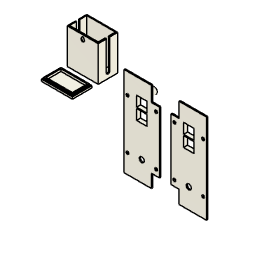
AP Panels (Autodesk Fusion 360 design; units mm, degrees)
Autodesk Fusion 360 part; units mm, degrees
sketch "Main" plane through (0, 0, 0) normal (0, 1, 0) x (1, 0, 0) in component "Front Left Plate"
  line L0 (-12, -11) -> (-12, 145)
  line L1 (-12, 145) -> (36, 145)
  line L2 (36, 145) -> (36, 122)
  line L3 (36, 122) -> (50, 122)
  line L4 (50, 122) -> (50, 15)
  line L5 (50, 15) -> (36, 15)
  line L6 (36, 15) -> (36, -11)
  line L7 (36, -11) -> (-12, -11)
  line L8 (-12, 0) -> (0, 0) construction
  line L9 (0, 0) -> (38, 0) construction
  line L10 (19, 145) -> (19, 139) construction
  line L11 (0, 139) -> (38, 139) construction
  line L12 (0, 139) -> (0, 0) construction
  line L13 (38, 139) -> (38, 0) construction
  line L14 (19, 139) -> (19, 0) construction
  circle A0 centre (-6, 25) radius 2.5
  line L15 (-6, 0) -> (-6, 139) construction
  line L16 (0, 139) -> (-12, 139) construction
  line L17 (36, 15) -> (-12, 15) construction
  line L18 (36, 122) -> (-12, 122) construction
  circle A1 centre (-6, 112) radius 2.5
  circle A2 centre (44, 25) radius 2.5
  circle A3 centre (44, 112) radius 2.5
  circle A4 centre (19, 110) radius 4.5
  line L19 (28, 55) -> (10, 55)
  line L20 (10, 55) -> (10, 37)
  line L21 (10, 37) -> (28, 37)
  line L22 (28, 37) -> (28, 55)
  line L23 (28, 55) -> (10, 37) construction
  line L24 (10, 55) -> (28, 37) construction
  line L25 (28, 35) -> (10, 35)
  line L26 (10, 35) -> (10, 17)
  line L27 (10, 17) -> (28, 17)
  line L28 (28, 17) -> (28, 35)
  line L29 (28, 35) -> (10, 17) construction
  line L30 (10, 35) -> (28, 17) construction
  point P0 (19, 46)
  point P1 (19, 26)
  dimension "d3" = 156
  dimension "d7" = 48
  dimension "d8" = 62
  dimension "d9" = 23
  dimension "d12" = 12
  dimension "d13" = 11
  dimension "d15" = 6
  dimension "d16" = 38
  dimension "d17" = 107
  dimension "d18" = 5
  dimension "d19" = 10
  dimension "d20" = 5
  dimension "d21" = 5
  dimension "d22" = 10
  dimension "d23" = 6
  dimension "d25" = 10
  dimension "d27" = 5
  dimension "d28" = 6
  dimension "d29" = 10
  dimension "d32" = 9
  dimension "d33" = 35
  dimension "d35" = 18
  dimension "d36" = 55
  dimension "d37" = 2
  constraint vertical L0
  constraint perpendicular L0 L1
  constraint perpendicular L2 L3
  constraint perpendicular L3 L4
  constraint perpendicular L4 L5
  constraint perpendicular L5 L6
  constraint horizontal L7
  constraint equal L1 L7
  constraint coincident L0 L8.start
  constraint perpendicular L0 L8
  constraint coincident L8.end L9.start
  constraint coincident L1 L10.start
  constraint perpendicular L1 L10
  constraint perpendicular L2 L11
  constraint midpoint L10.end L11
  constraint vertical L12
  constraint horizontal L9
  constraint equal L9 L11
  constraint midpoint L9 L14.end
  constraint midpoint L8 L15.start
  constraint perpendicular L8 L15
  constraint coincident L0 L16.end
  constraint perpendicular L0 L16
  constraint coincident L15.end L16
  constraint coincident A0.centre L15
  constraint coincident L0 L17.end
  constraint perpendicular L0 L17
  constraint coincident L0 L18.end
  constraint perpendicular L0 L18
  constraint coincident L15 A1.centre
  constraint coincident L14 A4.centre
  constraint horizontal L19
  constraint perpendicular L19 L20
  constraint parallel L19 L21
  constraint parallel L20 L22
  constraint coincident L23 P0
  constraint coincident L24 P0
  constraint coincident L14 P0
  constraint equal L19 L22
  constraint horizontal L25
  constraint perpendicular L25 L26
  constraint parallel L25 L27
  constraint parallel L26 L28
  constraint coincident L29 P1
  constraint coincident L30 P1
  constraint equal L22 L28
  constraint equal L22 L25
  constraint coincident L14 P1
  measures "d3" distance of L0.start L0.end
  measures "d7" distance of L0.end L1.end
  measures "d8" distance of L0 L4
  measures "d9" distance of L1.end L2.end
  measures "d12" distance of L8.start L8.end
  measures "d13" distance of L7 L8.end
  measures "d16" distance of L8.end L9.end
  measures "d17" distance of L3.end L4.end
  measures "d18" diameter of A0
  measures "d19" distance of A0.centre L17
  measures "d20" diameter of A1
  measures "d21" diameter of A2
  measures "d22" distance of L5 A2.centre
  measures "d23" distance of L4 A2.centre
  measures "d25" distance of L18 A1.centre
  measures "d27" diameter of A3
  measures "d28" distance of L4 A3.centre
  measures "d29" distance of L3 A3.centre
  measures "d32" diameter of A4
  measures "d33" distance of L1 A4.centre
  measures "d35" distance of L19.start L21.end
  measures "d36" distance of A4.centre L19
  measures "d37" distance of L21 L25
extrude "Extrude1" add sketch "Main" against normal blind 2 makes body 1 in component "Front Left Plate"
extrude "Extrude2" add sketch "Main" along normal blind 5 thin wall 2 outside contours L19 L20 L21 L22 | L25 L26 L27 L28 bodies 1 in component "Front Left Plate"
sketch "Sketch1" plane through (0, 0, 0) normal (0, 1, 0) x (1, 0, 0) in component "Button"
  line L0 (10.5, 17.5) -> (27.5, 17.5)
  line L1 (27.5, 17.5) -> (27.5, 34.5)
  line L2 (27.5, 34.5) -> (10.5, 34.5)
  line L3 (10.5, 34.5) -> (10.5, 17.5)
  line L4 (10.5, 17.5) -> (27.5, 34.5) construction
  line L5 (27.5, 17.5) -> (10.5, 34.5) construction
  point P0 (19, 26)
  point P1 (19, 26)
  dimension "d42" = 17
  constraint horizontal L0
  constraint perpendicular L0 L1
  constraint parallel L0 L2
  constraint parallel L1 L3
  constraint coincident L4 P1
  constraint coincident L5 P1
  constraint equal L0 L1
  constraint coincident P1 P0
  measures "d42" distance of L0.end L1.end
extrude "Extrude1'" add sketch "Sketch1" along normal blind 5 and the other way blind 3 separate body makes body 2 in component "Button"
sketch "Sketch2" plane through (0, 5, 0) normal (0, 1, 0) x (-1, 0, 0) in component "Button"
  line L0 (-10.5, -34.5) -> (-10.5, -17.5)
  line L1 (-10.5, -17.5) -> (-27.5, -17.5)
  line L2 (-27.5, -17.5) -> (-27.5, -34.5)
  line L3 (-27.5, -34.5) -> (-10.5, -34.5)
  line L4 (-8.5, -35.9) -> (-8.5, -15.5)
  line L5 (-8.5, -15.5) -> (-29.5, -15.5)
  line L6 (-29.5, -15.5) -> (-29.5, -35.9)
  line L7 (-29.5, -35.9) -> (-8.5, -35.9)
  dimension "d48" = 2
  dimension "d49" = 20.4
  constraint equal L4 L6
  measures "d49" distance of L4.start L4.end
extrude "Extrude2'" add sketch "Sketch2" along normal blind 2 contours L0 L1 L2 L3 | L4 L5 L6 L7 bodies 2 in component "Button"
sketch "Button Support" plane through (0, 0, 0) normal (0, 1, 0) x (-1, 0, 0) in component "Front Left Plate"
  line L0 (-30, -15) -> (-8, -15)
  line L1 (-8, -15) -> (-8, -57)
  line L2 (-8, -57) -> (-30, -57)
  line L3 (-30, -57) -> (-30, -15)
  circle A0 centre (6, -25) radius 2.5
  circle A1 centre (-44, -25) radius 2.5
  circle A2 centre (-19, -110) radius 4.5
  circle A3 centre (-44, -112) radius 2.5
  circle A4 centre (6, -112) radius 2.5
  line L4 (-36, 11) -> (-36, -15)
  line L5 (-36, -15) -> (-50, -15)
  line L6 (-50, -15) -> (-50, -122)
  line L7 (-50, -122) -> (-36, -122)
  line L8 (-36, -122) -> (-36, -145)
  line L9 (-36, -145) -> (12, -145)
  line L10 (12, -145) -> (12, 11)
  line L11 (12, 11) -> (-36, 11)
sketch "Board Support" plane through (0, 0, 0) normal (0, -1, 0) x (1, 0, 0) in component "Front Left Plate"
  circle A0 centre (-6, -25) radius 2.5
  line L0 (28, -17) -> (28, -35)
  line L1 (28, -35) -> (10, -35)
  line L2 (10, -35) -> (10, -17)
  line L3 (10, -17) -> (28, -17)
  circle A1 centre (44, -25) radius 2.5
  circle A2 centre (19, -110) radius 4.5
  line L4 (28, -37) -> (28, -55)
  line L5 (28, -55) -> (10, -55)
  line L6 (10, -55) -> (10, -37)
  line L7 (10, -37) -> (28, -37)
  circle A3 centre (44, -112) radius 2.5
  circle A4 centre (-6, -112) radius 2.5
  line L8 (36, -15) -> (36, 11)
  line L9 (36, 11) -> (-12, 11)
  line L10 (-12, 11) -> (-12, -145)
  line L11 (-12, -145) -> (36, -145)
  line L12 (36, -145) -> (36, -122)
  line L13 (36, -122) -> (50, -122)
  line L14 (50, -122) -> (50, -15)
  line L15 (50, -15) -> (36, -15)
  circle A5 centre (27, -8) radius 1.35
  circle A6 centre (27, -8) radius 5.3006
  circle A7 centre (11, -8) radius 1.35
  circle A8 centre (11, -8) radius 5.3006
  line L16 (27, -8) -> (11, -8) construction
  line L17 (19, -8) -> (19, 0) construction
  line L18 (30, -15) -> (8, -15)
  line L19 (8, -15) -> (8, -57)
  line L20 (8, -57) -> (30, -57)
  line L21 (30, -57) -> (30, -15)
  circle A9 centre (-6, -25) radius 2.5
  circle A10 centre (44, -25) radius 2.5
  circle A11 centre (19, -110) radius 4.5
  circle A12 centre (44, -112) radius 2.5
  circle A13 centre (-6, -112) radius 2.5
  line L22 (36, 11) -> (36, -15)
  line L23 (36, -15) -> (50, -15)
  line L24 (50, -15) -> (50, -122)
  line L25 (50, -122) -> (36, -122)
  line L26 (36, -122) -> (36, -145)
  line L27 (36, -145) -> (-12, -145)
  line L28 (-12, -145) -> (-12, 11)
  line L29 (-12, 11) -> (36, 11)
  line L30 (19, -8) -> (19, -84) construction
  circle A14 centre (27, -84) radius 5.3006
  circle A15 centre (27, -84) radius 1.35
  circle A16 centre (11, -84) radius 5.3006
  circle A17 centre (11, -84) radius 1.35
  line L31 (27, -84) -> (11, -84) construction
  point P0 (19, 0)
  dimension "d52" = 2.7
  dimension "d53" = 3.9506
  dimension "d54" = 3.9506
  dimension "d55" = 2.7
  dimension "d56" = 16
  dimension "d57" = 8
  dimension "d58" = 3.9506
  dimension "d59" = 3.9506
  dimension "d60" = 2.7
  dimension "d61" = 2.7
  dimension "d62" = 16
  dimension "d63" = 76
  constraint coincident A5.centre A6.centre
  constraint coincident A7.centre A8.centre
  constraint horizontal L16
  constraint parallel L8 L17
  constraint coincident P0 L17.end
  constraint midpoint L16 L17.start
  constraint perpendicular L20 L30
  constraint horizontal L31
  constraint midpoint L30.end L31
  constraint coincident A16.centre A17.centre
  constraint coincident A14.centre A15.centre
  measures "d52" diameter of A5
  measures "d55" diameter of A7
  measures "d56" distance of A5.centre A7.centre
  measures "d57" distance of L17.start P0
  measures "d60" diameter of A15
  measures "d61" diameter of A17
  measures "d62" distance of A16.centre A14.centre
  measures "d63" distance of L17.start L30.end
extrude "Extrude3" add sketch "Board Support" against normal blind 12 contours A6 | A8 | A14 | A16 bodies 1 in component "Front Left Plate"
sketch "Label Support" plane through (0, -2, 0) normal (0, -1, 0) x (1, 0, 0) in component "Front Left Plate"
  circle A0 centre (-6, -25) radius 2.5
  line L0 (28, -17) -> (28, -35)
  line L1 (28, -35) -> (10, -35)
  line L2 (10, -35) -> (10, -17)
  line L3 (10, -17) -> (28, -17)
  circle A1 centre (44, -25) radius 2.5
  circle A2 centre (19, -110) radius 4.5
  line L4 (28, -37) -> (28, -55)
  line L5 (28, -55) -> (10, -55)
  line L6 (10, -55) -> (10, -37)
  line L7 (10, -37) -> (28, -37)
  circle A3 centre (44, -112) radius 2.5
  circle A4 centre (-6, -112) radius 2.5
  line L8 (36, -15) -> (36, 11)
  line L9 (36, 11) -> (-12, 11)
  line L10 (-12, 11) -> (-12, -145)
  line L11 (-12, -145) -> (36, -145)
  line L12 (36, -145) -> (36, -122)
  line L13 (36, -122) -> (50, -122)
  line L14 (50, -122) -> (50, -15)
  line L15 (50, -15) -> (36, -15)
  line L16 (6, 5) -> (10, 5)
  line L17 (10, 5) -> (10, 3)
  line L18 (10, 3) -> (6, 3)
  line L19 (6, 3) -> (6, 5)
  line L20 (19, 4) -> (10, 4) construction
  line L21 (19, 0) -> (19, 11) construction
  line L22 (0, 0) -> (38, 0) construction
  line L23 (32, 3) -> (28, 3)
  line L24 (28, 3) -> (28, 5)
  line L25 (32, 5) -> (32, 3)
  line L26 (28, 5) -> (32, 5)
  line L27 (19, 4) -> (28, 4) construction
  line L28 (28, -137) -> (32, -137)
  line L29 (32, -137) -> (32, -139)
  line L30 (32, -139) -> (28, -139)
  line L31 (28, -139) -> (28, -137)
  line L32 (6, -137) -> (10, -137)
  line L33 (10, -137) -> (10, -139)
  line L34 (10, -139) -> (6, -139)
  line L35 (6, -139) -> (6, -137)
  line L36 (8, -137) -> (8, 3) construction
  line L37 (30, -137) -> (30, 3) construction
  line L38 (8, -139) -> (8, -145) construction
  line L39 (30, -139) -> (30, -145) construction
  dimension "d67" = 38
  dimension "d68" = 2
  dimension "d69" = 4
  dimension "d70" = 4
  dimension "d71" = 9
  dimension "d73" = 6
  dimension "d74" = 6
  constraint horizontal L16
  constraint vertical L17
  constraint horizontal L18
  constraint vertical L19
  constraint coincident L17 L20.end
  constraint perpendicular L17 L20
  constraint coincident L9 L21.end
  constraint perpendicular L9 L21
  constraint coincident L20.start L21
  constraint perpendicular L8 L22
  constraint coincident L22.start origin
  constraint midpoint L21.start L22
  constraint horizontal L26
  constraint vertical L25
  constraint horizontal L23
  constraint vertical L24
  constraint equal L19 L24
  constraint equal L18 L23
  constraint midpoint L24 L27.end
  constraint equal L20 L27
  constraint horizontal L27
  constraint midpoint L17 L20.end
  constraint horizontal L28
  constraint vertical L29
  constraint horizontal L30
  constraint vertical L31
  constraint horizontal L32
  constraint vertical L33
  constraint horizontal L34
  constraint vertical L35
  constraint equal L19 L35
  constraint equal L19 L31
  constraint equal L18 L34
  constraint equal L23 L30
  constraint midpoint L32 L36.start
  constraint midpoint L18 L36.end
  constraint midpoint L28 L37.start
  constraint midpoint L23 L37.end
  constraint equal L36 L37
  constraint vertical L36
  constraint vertical L37
  constraint midpoint L34 L38.start
  constraint coincident L11 L38.end
  constraint perpendicular L11 L38
  constraint midpoint L30 L39.start
  constraint coincident L11 L39.end
  constraint perpendicular L11 L39
  measures "d67" distance of L22.start L22.end
  measures "d68" distance of L16.start L18.end
  measures "d69" distance of L16.start L16.end
  measures "d70" distance of L20 L22
  measures "d71" distance of L20.start L20.end
  measures "d73" distance of L9 L26
  measures "d74" distance of L38.start L38.end
mirror "Mirror1" about plane through (0, 0, 0) normal (1, 0, 0) of bodies 1 makes body 3 in component "Front Left Plate"
move_body "Move1" bodies 3 to x (1, 0, 0) y (0, 1, 0) z (0, 0, 1) at (120, 0, 0) in component "Front Left Plate"
sketch "Main Case" plane through (0, 0, 0) normal (0, 0, 1) x (1, 0, 0) in component "Arduino Case"
  line L0 (-25, 0) -> (-79, 0)
  line L1 (-79, 0) -> (-79, -34)
  line L2 (-79, -34) -> (-25, -34)
  line L3 (-25, -34) -> (-25, 0)
  line L4 (0, 0) -> (-25, 0) construction
  line L5 (-54.5, -5) -> (-49.5, -5)
  line L6 (-49.5, -13) -> (-54.5, -13)
  line L7 (-52, 0) -> (-52, -5) construction
  arc A0 (-54.5, -5) -> (-54.5, -13) centre (-54.5, -9) ccw
  arc A1 (-49.5, -13) -> (-49.5, -5) centre (-49.5, -9) ccw
  line L8 (-58.5, -9) -> (-45.5, -9) construction
  dimension "d95" = 54
  dimension "d96" = 34
  dimension "d106" = 25
  dimension "d116" = 8
  dimension "d118" = 5
  dimension "d119" = 13
  constraint horizontal L0
  constraint vertical L1
  constraint horizontal L2
  constraint vertical L3
  constraint coincident L4.start origin
  constraint perpendicular L3 L4
  constraint equal A0 A1
  constraint tangent L5 A1
  constraint parallel L0 L5
  constraint tangent L6 A0
  constraint parallel L5 L6
  constraint equal L5 L6
  constraint midpoint L0 L7.start
  constraint perpendicular L0 L7
  constraint midpoint L5 L7.end
  constraint midpoint A0 L8.start
  constraint midpoint A1 L8.end
  constraint tangent L6 A1
  measures "d95" distance of L1.end L2.end
  measures "d96" distance of L0.end L1.end
  measures "d106" distance of L0.start L4.start
  measures "d116" diameter of A0
  measures "d118" distance of L7.start L7.end
  measures "d119" horizontal distance of L8.start L8.end
extrude "Extrude1''" add sketch "Main Case" against normal blind 2 separate body contours L0 L1 L2 L3 | L5 L6 A0 A1 makes body 4 in component "Arduino Case"
extrude "Extrude2''" add 1 faces at (-43, -22.6667, 0) along direction (0, 0, 1) blind 60 thin wall 2 inside on bodies 4 bodies 4 in component "Arduino Case"
sketch "Side Hole" plane through (-79, 0, 0) normal (-1, 0, 0) x (0, -1, 0) in component "Arduino Case"
  line L0 (0, 60) -> (0, -2)
  line L1 (0, -2) -> (34, -2)
  line L2 (34, -2) -> (34, 60)
  line L3 (34, 60) -> (0, 60)
  line L4 (17, -2) -> (17, 8) construction
  circle A0 centre (17, 8) radius 2.5
  line L5 (19.5, 8) -> (19.5, 60)
  line L6 (14.5, 8) -> (14.5, 60)
  dimension "d104" = 5
  dimension "d105" = 10
  constraint midpoint L1 L4.start
  constraint perpendicular L1 L4
  constraint coincident L4.end A0.centre
  constraint coincident A0 L5.start
  constraint coincident L3 L5.end
  constraint perpendicular L3 L5
  constraint coincident A0 L6.start
  constraint coincident L3 L6.end
  constraint perpendicular L3 L6
  constraint tangent A0 L6
  constraint tangent A0 L5
  measures "d104" diameter of A0
  measures "d105" distance of L4.start L4.end
extrude "Extrude3'" cut sketch "Side Hole" against normal through all contours L3 A0 L5 L6 | A0 bodies 4 in component "Arduino Case"
chamfer "Chamfer1" distance 0.5 angle 45 6 edges at (-52, -34, 60) (-25, -26.75, 60) (-25, -7.25, 60) (-52, 0, 60) (-79, -7.25, 60) (-79, -26.75, 60) on bodies 4 in component "Arduino Case"
sketch "Mounting Hole" plane through (0, -34, 0) normal (0, -1, 0) x (1, 0, 0) in component "Arduino Case"
  line L0 (-25, 59.5) -> (-79, 59.5)
  line L1 (-79, 59.5) -> (-79, -2)
  line L2 (-79, -2) -> (-25, -2)
  line L3 (-25, -2) -> (-25, 59.5)
  line L4 (-52, 59.5) -> (-52, 51.5) construction
  line L5 (-52, 51.5) -> (-52, 54.5) construction
  line L6 (-54, 54.5) -> (-54, 54.1458)
  line L7 (-50, 54.5) -> (-50, 54.1458)
  arc A0 (-54.25, 53.4843) -> (-49.75, 53.4843) centre (-52, 51.5) ccw
  arc A1 (-54.25, 53.4843) -> (-54, 54.1458) centre (-55, 54.1458) ccw
  arc A2 (-50, 54.1458) -> (-49.75, 53.4843) centre (-49, 54.1458) ccw
  arc A3 (-50, 54.5) -> (-54, 54.5) centre (-52, 54.5) ccw
  dimension "d109" = 6
  dimension "d110" = 8
  dimension "d111" = 4
  dimension "d112" = 3
  dimension "d113" = 1
  constraint midpoint L0 L4.start
  constraint perpendicular L0 L4
  constraint coincident L4.end L5.start
  constraint coincident L4 L5.end
  constraint coincident L5.end A3.centre
  constraint parallel L5 L6
  constraint parallel L5 L7
  constraint tangent L7 A3
  constraint tangent L6 A3
  constraint tangent L6 A1
  constraint tangent A0 A1
  constraint tangent L7 A2
  constraint tangent A0 A2
  constraint equal A1 A2
  measures "d109" diameter of A0
  measures "d110" distance of L4.start L4.end
  measures "d111" diameter of A3
  measures "d112" distance of L4.end L5.end
  measures "d113" radius of A1
extrude "Extrude4" cut sketch "Mounting Hole" against normal up to surface (2 mm away) contours L6 L7 A0 A1 A2 A3 bodies 4 in component "Arduino Case"
extrude "Extrude5" cut sketch "Main Case" against normal up to surface (2 mm away) contours L5 L6 A0 A1 bodies 4 in component "Arduino Case"
chamfer "Chamfer2" distance 1 angle 45 6 edges at (-52, -32, 56.5) (-54, -32, 54.3229) (-54.0646, -32, 53.7922) (-52, -32, 48.5) (-49.9354, -32, 53.7922) (-50, -32, 54.3229) on bodies 4 in component "Arduino Case"
fillet "Fillet1" radius 0.5 12 edges at (-27, -19.5, 34) (-27, -17, 5.5) (-27, -14.5, 34) (-77, -14.5, 34) (-77, -17, 5.5) (-77, -19.5, 34) (-79, -19.5, 33.75) (-79, -17, 5.5) (-79, -14.5, 33.75) (-25, -14.5, 33.75) (-25, -17, 5.5) (-25, -19.5, 33.75) on bodies 4 in component "Arduino Case"
sketch "Cover" plane through (0, 0, 0) normal (0, 0, 1) x (1, 0, 0) in component "Arduino Case Cover"
  line L0 (-79, -45) -> (-25, -45)
  line L1 (-25, -45) -> (-25, -79)
  line L2 (-25, -79) -> (-79, -79)
  line L3 (-79, -79) -> (-79, -45)
  line L4 (-79, -34) -> (-25, -34)
  line L5 (-79, 0) -> (-79, -34)
  line L6 (0, -45) -> (-25, -45) construction
  line L7 (0, 0) -> (0, -45) construction
  line L8 (0, 0) -> (-25, 0) construction
  line L9 (-27, -77) -> (-77, -77)
  line L10 (-77, -77) -> (-77, -47)
  line L11 (-77, -47) -> (-27, -47)
  line L12 (-27, -47) -> (-27, -77)
  line L13 (-29, -75) -> (-75, -75)
  line L14 (-75, -75) -> (-75, -49)
  line L15 (-75, -49) -> (-29, -49)
  line L16 (-29, -49) -> (-29, -75)
  dimension "d125" = 45
  dimension "d131" = 2
  dimension "d132" = 4
  constraint horizontal L0
  constraint vertical L1
  constraint horizontal L2
  constraint vertical L3
  constraint equal L0 L4
  constraint equal L3 L5
  constraint perpendicular L1 L6
  constraint coincident L0.end L1.start
  constraint coincident L7.start L8.start
  constraint vertical L7
  constraint coincident L6.start L7.end
  constraint equal L6 L8
  measures "d125" distance of L7.start L6.start
extrude "Extrude1'''" add sketch "Cover" against normal blind 2 separate body contours L0 L1 L2 L3 | L9 L10 L11 L12 | L13 L14 L15 L16 makes body 5 in component "Arduino Case Cover"
extrude "Extrude3''" add sketch "Cover" along normal blind 2 contours L0 L1 L2 L3 | L9 L10 L11 L12 bodies 5 in component "Arduino Case Cover"
extrude "Extrude4'" add sketch "Cover" along normal blind 4 contours L9 L10 L11 L12 bodies 5 in component "Arduino Case Cover"
chamfer "Chamfer1'" distance 0.5 angle 45 4 edges at (-52, -79, 2) (-25, -62, 2) (-79, -62, 2) (-52, -45, 2) on bodies 5 in component "Arduino Case Cover"
component "Front Left Plate" placed x (1, 0, 0) y (0, 1, 0) z (0, 0, 1) at (0, 0, 0)
component "Button" placed x (1, 0, 0) y (0, 1, 0) z (0, 0, 1) at (0, 0, 0)
component "Arduino Case" placed x (1, 0, 0) y (0, 1, 0) z (0, 0, 1) at (0, 0, 0)
component "Arduino Case Cover" placed x (1, 0, 0) y (0, 1, 0) z (0, 0, 1) at (0, 0, 0)
equation "d22 = d19"
equation "d25 = d19"
equation "d28 = d23"
equation "d29 = d19"
equation "d35 = ButtonHoleEdgeLength"
equation "ButtonHoleEdgeLength = 18 mm"
equation "d42 = ButtonHoleEdgeLength - 1 mm"
equation "d49 = d48 + ButtonHoleEdgeLength + 0.4 mm"
equation "d67 = d16"
equation "d74 = d73"
named bodies: "Case"
